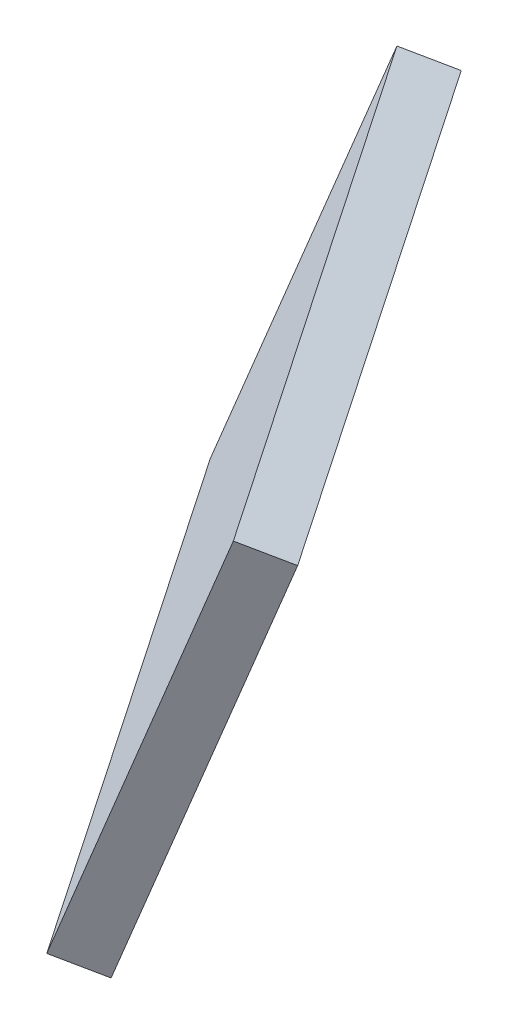
# Autodesk Inventor part: Część9
Saved by Autodesk Inventor 2025.1 (Build 291241020, 241B)
## iProperties
Created: 2024-10-13
Part Number: Część9
Material: Ogólny
Document SubType Name: Modeling
Designer: zychlix
Density: 1 g/cm^3
Appearance: Domyślna
Author: zychlix
Autodesk Inventor part; units mm, degrees
ref_plane "YZ Plane" through (0, 0, 0) normal (1, 0, 0) x (0, 1, 0)
ref_plane "XZ Plane" through (0, 0, 0) normal (0, 1, 0) x (-1, 0, 0)
ref_plane "XY Plane" through (0, 0, 0) normal (0, 0, 1) x (1, 0, 0)
ref_plane "Płaszczyzna konstrukcyjna1" through (49.6691, -19.5986, -3) normal (0.3827, 0.9239, 0) x (-0.9239, 0.3827, 0)
sketch "Szkic1" plane through (49.6691, -19.5986, -3) normal (0.3827, 0.9239, 0) x (-0.9239, 0.3827, 0)
  line L0 (0, 0) -> (66.0187, 0) construction
  line L1 (53.7615, 0) -> (97.5647, 28.4461) construction
  line L2 (53.7615, 0) -> (72.5205, 42.1334) construction
  line L3 (0, 0) -> (66.0187, 0) construction
  point P0 (53.3884, 3)
  point P1 (71.7596, 40.4245)
  dimension "d0" = 33
  dimension "d1" = 66
  constraints: 4 end point, 1 point on line
  measures "d0" angle of L1 L0
  measures "d1" angle of L2 L0
ref_plane "Płaszczyzna konstrukcyjna2" through (-16.6281, 7.8626, 37.4245) normal (-0.7748, 0.3209, 0.5446) x (-0.3827, -0.9239, 0)
ref_plane "Płaszczyzna konstrukcyjna3" through (0, 0, 0) normal (0, 0, 1) x (1, 0, 0)
sketch "Szkic2" plane through (0, 0, 0) normal (0, 0, 1) x (1, 0, 0)
  point P0 (0, 0)
sketch "Szkic3" plane through (-16.6281, 7.8626, 37.4245) normal (-0.7748, 0.3209, 0.5446) x (-0.3827, -0.9239, 0)
  line L0 (10.7362, 10.6866) -> (-9.2638, 10.6866)
  line L1 (-9.2638, 10.6866) -> (-9.2638, -9.3134)
  line L2 (-9.2638, -9.3134) -> (10.7362, -9.3134)
  line L3 (10.7362, -9.3134) -> (10.7362, 10.6866)
  point P0 (0.9008, -21.3811)
  dimension "d2" = 20
  dimension "d3" = 20
  constraints: 8 end point, 2 parallel, 1 horizontal, 1 perpendicular
  measures "d2" distance of L2.end L0.start
  measures "d3" distance of L1.end L2.end
extrude "Wyciągnięcie proste1" add sketch "Szkic3" along normal blind 2
